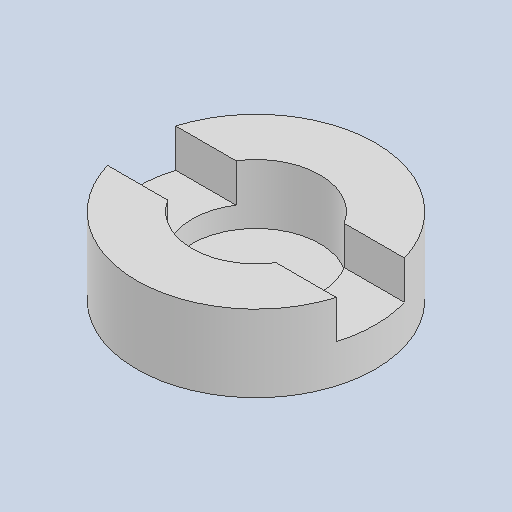
# Autodesk Inventor part: magneticslotV1
Saved by Autodesk Inventor 2022.1 (Build 261234020, 234B)
## iProperties
Created: 2021-06-03
Part Number: magneticslotV1
Material: Generic
Document SubType Name: Modeling
Designer: User
Density: 1 g/cm^3
Appearance: Default
Author: User
Autodesk Inventor part; units mm, degrees
ref_plane "YZ Plane" through (0, 0, 0) normal (1, 0, 0) x (0, 1, 0)
ref_plane "XZ Plane" through (0, 0, 0) normal (0, 1, 0) x (-1, 0, 0)
ref_plane "XY Plane" through (0, 0, 0) normal (0, 0, 1) x (1, 0, 0)
sketch "Sketch1" plane through (0, 0, 0) normal (0, 1, 0) x (-1, 0, 0)
  circle A0 centre (0, 0) radius 14
  circle A1 centre (0, 0) radius 7.5
  dimension "d0" = 28
  dimension "d1" = 15
  constraints: 2 centre point, 2 coincident
  measures "d0" diameter of A0
  measures "d1" diameter of A1
extrude "Extrusion1" add sketch "Sketch1" along normal blind 7
sketch "Sketch2" plane through (0, 7, 0) normal (0, 1, 0) x (1, 0, 0)
  line L0 (14, -4) -> (-14, -4)
  line L1 (-14, -4) -> (-14, 4)
  line L2 (-14, 4) -> (14, 4)
  line L3 (14, 4) -> (14, -4)
  line L4 (14, -4) -> (-14, 4) construction
  line L5 (-14, -4) -> (14, 4) construction
  line L6 (-0.5, 5) -> (0.5, 5)
  line L7 (0.5, 5) -> (0.5, -5)
  line L8 (0.5, -5) -> (-0.5, -5)
  line L9 (-0.5, -5) -> (-0.5, 5)
  line L10 (-0.5, 5) -> (0.5, -5) construction
  line L11 (0.5, 5) -> (-0.5, -5) construction
  point P0 (0, 0)
  dimension "d4" = 28
  dimension "d5" = 8
  constraints: 24 end point, 4 midpoint, 4 parallel, 2 horizontal, 2 perpendicular
  measures "d4" distance of L1.end L2.end
  measures "d5" distance of L0.end L1.end
extrude "Extrusion2" cut sketch "Sketch2" against normal blind 8 contours L0 L7 L2 L3 | L0 L9 L2 L7 | L0 L1 L2 L9
sketch "Sketch3" plane through (0, 0, 0) normal (0, -1, 0) x (1, 0, 0)
  circle A0 centre (0, 0) radius 14
  dimension "d17" = 28
  constraints: 1 centre point, 1 coincident
  measures "d17" diameter of A0
extrude "Extrusion3" add sketch "Sketch3" along normal blind 2
sketch "Sketch5" plane through (0, 0, 0) normal (0, 1, 0) x (1, 0, 0)
  point P0 (0, 0)
  point P1 (-0.0372, -0.1116)
hole "Hole2" at (-0.0372, 0, 0.1116) direction (0, -1, 0) diameter 4.5 end through all clearance for "Hex Head Machine Screw" size "M4" standard "Ansi Metric M Profile"
extrude "Extrusion4" add sketch "Sketch1" along normal blind 2.5
body "Solid1"
